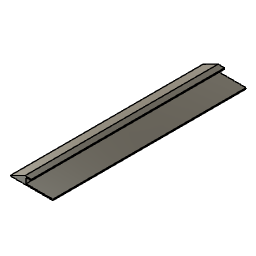
trim-right v3 (Autodesk Fusion 360 design; units mm, degrees)
Autodesk Fusion 360 part; units mm, degrees
sketch "Sketch1" plane through (0, 0, 0) normal (0, 1, 0) x (1, 0, 0)
  line L0 (-30, 0) -> (10, 0)
  line L1 (10, 0) -> (10, -1)
  line L2 (10, -1) -> (-15, -1)
  line L3 (-15, -1) -> (-15, -6)
  line L4 (-15, -6) -> (-10, -6)
  line L5 (-10, -6) -> (-10, -7)
  line L6 (-10, -7) -> (-16, -7)
  line L7 (-16, -7) -> (-30, 0)
  dimension "d1" = 40
  dimension "d2" = 1
  constraint horizontal L0
  constraint vertical L1
  constraint perpendicular L1 L2
  constraint perpendicular L2 L3
  constraint perpendicular L3 L4
  constraint perpendicular L4 L5
  constraint perpendicular L3 L6
  measures "d1" distance of L0.start L0.end
  measures "d2" distance of L0.end L1.end
sketch "Sketch2" plane through (0, 0, 0) normal (0, 1, 0) x (1, 0, 0)
extrude "Extrude1" add sketch "Sketch1" along normal blind 200
sketch "Sketch3" plane through (0, 0, 0) normal (0, -1, 0) x (1, 0, 0)
  line L0 (-10, 7) -> (-16, 7)
  line L1 (-16, 7) -> (-30, 0)
  line L2 (-30, 0) -> (10, 0)
  line L3 (10, 0) -> (10, 1)
  line L4 (10, 1) -> (-15, 1)
  line L5 (-15, 1) -> (-15, 6)
  line L6 (-15, 6) -> (-10, 6)
  line L7 (-10, 6) -> (-10, 7)
  circle A0 centre (-18, 3) radius 1.5
  dimension "d5" = 3
  dimension "d6" = 3
  dimension "d7" = 3
  measures "d5" diameter of A0
  measures "d6" distance of L5 A0.centre
  measures "d7" distance of L2 A0.centre
extrude "Extrude2" add sketch "Sketch3" along normal blind 10 contours A0
sketch "Sketch4" plane through (0, 0, 0) normal (0, 1, 0) x (1, 0, 0)
sketch "Sketch5" plane through (0, 200, 0) normal (0, 1, 0) x (-1, 0, 0)
  line L0 (16, 7) -> (10, 7)
  line L1 (10, 7) -> (10, 6)
  line L2 (10, 6) -> (15, 6)
  line L3 (15, 6) -> (15, 1)
  line L4 (15, 1) -> (-10, 1)
  line L5 (-10, 1) -> (-10, 0)
  line L6 (-10, 0) -> (30, 0)
  line L7 (30, 0) -> (16, 7)
  circle A0 centre (18, 3) radius 1.5
  dimension "d10" = 3
  dimension "d11" = 3
  dimension "d12" = 3
  measures "d10" diameter of A0
  measures "d11" distance of L6 A0.centre
  measures "d12" distance of L3 A0.centre
extrude "Extrude3" cut sketch "Sketch5" against normal blind 11 contours A0
delete_face "DeleteFace1" 1 faces at (-16.5019, -6.6667, 2.9252)
extrude "Extrude4" cut 1 faces at (-20.3333, 0, 2.6667) along direction (0, 1, 0) blind 20
